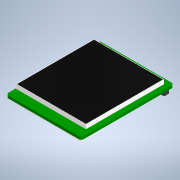
# Autodesk Inventor part: Display
Saved by Autodesk Inventor 2020 (Build 240168000, 168)
## iProperties
Created: 2021-03-29
Part Number: Display
Material: Generic
Document SubType Name: Modeling
Designer: Luke
Density: 1 g/cm^3
Appearance: Default
Author: Luke
Autodesk Inventor part; units mm, degrees
ref_plane "YZ Plane" through (0, 0, 0) normal (1, 0, 0) x (0, 1, 0)
ref_plane "XZ Plane" through (0, 0, 0) normal (0, 1, 0) x (-1, 0, 0)
ref_plane "XY Plane" through (0, 0, 0) normal (0, 0, 1) x (1, 0, 0)
sketch "Sketch1" plane through (0, 0, 0) normal (0, 1, 0) x (-1, 0, 0)
  line L0 (16.25, 21) -> (-16.25, 21)
  line L1 (-17.05, 20.2) -> (-17.05, -20.2)
  line L2 (-16.25, -21) -> (16.25, -21)
  line L3 (17.05, -20.2) -> (17.05, 20.2)
  line L4 (17.05, 21) -> (-17.05, -21) construction
  line L5 (-17.05, 21) -> (17.05, -21) construction
  line L6 (16.25, 21) -> (17.05, 20.2)
  line L7 (17.05, -20.2) -> (16.25, -21)
  line L8 (-16.25, -21) -> (-17.05, -20.2)
  line L9 (-17.05, 20.2) -> (-16.25, 21)
  point P0 (0, 0)
  dimension "d0" = 34.1
  dimension "d1" = 42
  dimension "d4" = 0.8
  dimension "d5" = 0.8
  dimension "d6" = 0.8
  dimension "d7" = 0.8
  dimension "d8" = 0.8
  dimension "d9" = 0.8
  dimension "d10" = 0.8
  dimension "d11" = 0.8
  constraints: 20 end point, 8 point on line, 2 midpoint, 2 parallel, 1 horizontal, 1 perpendicular
  measures "d0" distance of L5.end L4.end
  measures "d1" distance of L4.end L5.start
  measures "d4" distance of L0.start L4.start
  measures "d5" distance of L3.end L4.start
  measures "d6" distance of L3.start L5.end
  measures "d7" distance of L2.end L5.end
  measures "d8" distance of L2.start L4.end
  measures "d9" distance of L1.end L4.end
  measures "d10" distance of L1.start L5.start
  measures "d11" distance of L0.end L5.start
extrude "Extrusion1" add sketch "Sketch1" along normal blind 1.2
ref_plane "Work Plane1" through (0, 2.2, 0) normal (0, 1, 0) x (1, 0, 0)
sketch "Sketch2" plane through (0, 2.2, 0) normal (0, 1, 0) x (1, 0, 0)
  line L0 (-15.85, -17.675) -> (15.85, -17.675)
  line L1 (15.85, -17.675) -> (15.85, 17.675)
  line L2 (15.85, 17.675) -> (-15.85, 17.675)
  line L3 (-15.85, 17.675) -> (-15.85, -17.675)
  line L4 (-15.85, -17.675) -> (15.85, 17.675) construction
  line L5 (15.85, -17.675) -> (-15.85, 17.675) construction
  point P0 (0, 0)
  dimension "d13" = 31.7
  dimension "d14" = 35.35
  constraints: 12 end point, 2 midpoint, 2 parallel, 1 horizontal, 1 perpendicular
  measures "d13" distance of L2.end L1.end
  measures "d14" distance of L1.end L0.end
extrude "Extrusion2" add sketch "Sketch2" along normal blind 1.8
sketch "Sketch3" plane through (0, 4, 0) normal (0, 1, 0) x (1, 0, 0)
  line L0 (-15.85, -17.675) -> (15.85, -17.675) projected
  line L1 (15.85, -17.675) -> (15.85, 17.675) projected
  line L2 (15.85, 17.675) -> (-15.85, 17.675) projected
  line L3 (-15.85, 17.675) -> (-15.85, -17.675) projected
  line L4 (-15.65, -17.475) -> (15.65, -17.475)
  line L5 (15.65, -17.475) -> (15.65, 17.475)
  line L6 (15.65, 17.475) -> (-15.65, 17.475)
  line L7 (-15.65, 17.475) -> (-15.65, -17.475)
  point P0 (0, 0)
  dimension "d17" = 0.2
  constraints: 8 end point, 3 other
  measures "d17" distance between parallel lines of L3 L7
extrude "Extrusion3" add sketch "Sketch3" along normal blind 0.1
sketch "Sketch4" plane through (0, 1.2, 0) normal (0, 1, 0) x (1, 0, 0)
  line L0 (-14, -10) -> (14, -10)
  line L1 (14, -10) -> (14, 10)
  line L2 (14, 10) -> (-14, 10)
  line L3 (-14, 10) -> (-14, -10)
  line L4 (-14, -10) -> (14, 10) construction
  line L5 (14, -10) -> (-14, 10) construction
  point P0 (0, 0)
  dimension "d20" = 28
  dimension "d21" = 20
  constraints: 12 end point, 2 midpoint, 2 parallel, 1 horizontal, 1 perpendicular
  measures "d20" distance of L2.end L1.end
  measures "d21" distance of L1.end L0.end
extrude "Extrusion4" add sketch "Sketch4" along normal up to surface (1 mm away)
sketch "Sketch5" plane through (0, 0, 0) normal (0, -1, 0) x (1, 0, 0)
  line L0 (15.8, -20) -> (13.86, -20)
  line L1 (13.61, -19.75) -> (13.61, -17.81)
  line L2 (13.86, -17.56) -> (15.8, -17.56)
  line L3 (16.05, -17.81) -> (16.05, -19.75)
  line L4 (16.05, -19.75) -> (15.8, -20)
  line L5 (13.86, -20) -> (13.61, -19.75)
  line L6 (13.61, -17.81) -> (13.86, -17.56)
  line L7 (15.8, -17.56) -> (16.05, -17.81)
  line L8 (13.36, -20) -> (11.42, -20)
  line L9 (11.17, -19.75) -> (11.17, -17.81)
  line L10 (11.42, -17.56) -> (13.36, -17.56)
  line L11 (13.61, -17.81) -> (13.61, -19.75)
  line L12 (13.61, -19.75) -> (13.36, -20)
  line L13 (11.42, -20) -> (11.17, -19.75)
  line L14 (11.17, -17.81) -> (11.42, -17.56)
  line L15 (13.36, -17.56) -> (13.61, -17.81)
  line L16 (10.92, -20) -> (8.98, -20)
  line L17 (8.73, -19.75) -> (8.73, -17.81)
  line L18 (8.98, -17.56) -> (10.92, -17.56)
  line L19 (11.17, -17.81) -> (11.17, -19.75)
  line L20 (11.17, -19.75) -> (10.92, -20)
  line L21 (8.98, -20) -> (8.73, -19.75)
  line L22 (8.73, -17.81) -> (8.98, -17.56)
  line L23 (10.92, -17.56) -> (11.17, -17.81)
  line L24 (8.48, -20) -> (6.54, -20)
  line L25 (6.29, -19.75) -> (6.29, -17.81)
  line L26 (6.54, -17.56) -> (8.48, -17.56)
  line L27 (8.73, -17.81) -> (8.73, -19.75)
  line L28 (8.73, -19.75) -> (8.48, -20)
  line L29 (6.54, -20) -> (6.29, -19.75)
  line L30 (6.29, -17.81) -> (6.54, -17.56)
  line L31 (8.48, -17.56) -> (8.73, -17.81)
  line L32 (6.04, -20) -> (4.1, -20)
  line L33 (3.85, -19.75) -> (3.85, -17.81)
  line L34 (4.1, -17.56) -> (6.04, -17.56)
  line L35 (6.29, -17.81) -> (6.29, -19.75)
  line L36 (6.29, -19.75) -> (6.04, -20)
  line L37 (4.1, -20) -> (3.85, -19.75)
  line L38 (3.85, -17.81) -> (4.1, -17.56)
  line L39 (6.04, -17.56) -> (6.29, -17.81)
  line L40 (3.6, -20) -> (1.66, -20)
  line L41 (1.41, -19.75) -> (1.41, -17.81)
  line L42 (1.66, -17.56) -> (3.6, -17.56)
  line L43 (3.85, -17.81) -> (3.85, -19.75)
  line L44 (3.85, -19.75) -> (3.6, -20)
  line L45 (1.66, -20) -> (1.41, -19.75)
  line L46 (1.41, -17.81) -> (1.66, -17.56)
  line L47 (3.6, -17.56) -> (3.85, -17.81)
  line L48 (1.16, -20) -> (-0.78, -20)
  line L49 (-1.03, -19.75) -> (-1.03, -17.81)
  line L50 (-0.78, -17.56) -> (1.16, -17.56)
  line L51 (1.41, -17.81) -> (1.41, -19.75)
  line L52 (1.41, -19.75) -> (1.16, -20)
  line L53 (-0.78, -20) -> (-1.03, -19.75)
  line L54 (-1.03, -17.81) -> (-0.78, -17.56)
  line L55 (1.16, -17.56) -> (1.41, -17.81)
  line L56 (-1.28, -20) -> (-3.22, -20)
  line L57 (-3.47, -19.75) -> (-3.47, -17.81)
  line L58 (-3.22, -17.56) -> (-1.28, -17.56)
  line L59 (-1.03, -17.81) -> (-1.03, -19.75)
  line L60 (-1.03, -19.75) -> (-1.28, -20)
  line L61 (-3.22, -20) -> (-3.47, -19.75)
  line L62 (-3.47, -17.81) -> (-3.22, -17.56)
  line L63 (-1.28, -17.56) -> (-1.03, -17.81)
  point P0 (16.05, -20)
  point P1 (13.61, -17.56)
  point P2 (13.61, -20)
  point P3 (16.05, -17.56)
  point P4 (13.61, -20)
  point P5 (11.17, -17.56)
  point P6 (11.17, -20)
  point P7 (13.61, -17.56)
  point P8 (11.17, -20)
  point P9 (8.73, -17.56)
  point P10 (8.73, -20)
  point P11 (11.17, -17.56)
  point P12 (8.73, -20)
  point P13 (6.29, -17.56)
  point P14 (6.29, -20)
  point P15 (8.73, -17.56)
  point P16 (6.29, -20)
  point P17 (3.85, -17.56)
  point P18 (3.85, -20)
  point P19 (6.29, -17.56)
  point P20 (3.85, -20)
  point P21 (1.41, -17.56)
  point P22 (1.41, -20)
  point P23 (3.85, -17.56)
  point P24 (1.41, -20)
  point P25 (-1.03, -17.56)
  point P26 (-1.03, -20)
  point P27 (1.41, -17.56)
  point P28 (-1.03, -20)
  point P29 (-3.47, -17.56)
  point P30 (-3.47, -20)
  point P31 (-1.03, -17.56)
  dimension "d42" = 2.44
  constraints: 128 end point, 64 point on line, 2 horizontal, 2 parallel, 1 collinear, 1 perpendicular, 139 other
  measures "d42" distance of point (16.05, -20) point (13.61, -20)
extrude "Extrusion5" add sketch "Sketch5" along normal blind 2.44
sketch "Sketch6" plane through (0, 0, 0) normal (0, -1, 0) x (1, 0, 0)
  line L0 (-15, 8.95) -> (15, 8.95)
  line L1 (15, 8.95) -> (15, 18.95)
  line L2 (15, 18.95) -> (-15, 18.95)
  line L3 (-15, 18.95) -> (-15, 8.95)
  line L4 (-15, 8.95) -> (15, 18.95) construction
  line L5 (15, 8.95) -> (-15, 18.95) construction
  line L6 (-16.25, 21) -> (16.25, 21) projected
  line L7 (0, 21) -> (0, 18.95)
  point P0 (0, 0)
  point P1 (0, 18.95)
  dimension "d49" = 30
  dimension "d50" = 10
  dimension "d51" = 2.05
  constraints: 14 end point, 2 midpoint, 2 parallel, 1 horizontal, 1 perpendicular, 1 vertical
  measures "d49" distance of L2.end L1.end
  measures "d50" distance of L1.end L0.end
  measures "d51" distance of L7.start L7.end
ref_plane "Work Plane2" through (-19.708, -2.44, -51.7905) normal (0, 1, 0) x (0, 0, 1)
extrude "Extrusion6" add sketch "Sketch6" along normal up to surface (2.44 mm away)
equation "\"d5\" = d4"
equation "\"d6\" = d4"
equation "\"d7\" = d6"
equation "\"d8\" = d4"
equation "\"d9\" = d8"
equation "\"d10\" = d4"
equation "\"d11\" = d10"
body "Solid1"
